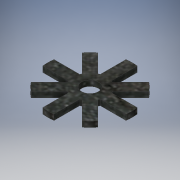
# Autodesk Inventor part: Tooth Disc
Saved by Autodesk Inventor 2019 (Build 230136000, 136)
## iProperties
Created: 2020-01-31
Part Number: Tooth Disc
Material: Steel
Document SubType Name: Modeling
Designer: alb16148
Density: 7.85 g/cm^3
Appearance: Plate
Author: alb16148
Autodesk Inventor part; units mm, degrees
ref_plane "YZ Plane" through (0, 0, 0) normal (1, 0, 0) x (0, 1, 0)
ref_plane "XZ Plane" through (0, 0, 0) normal (0, 1, 0) x (-1, 0, 0)
ref_plane "XY Plane" through (0, 0, 0) normal (0, 0, 1) x (1, 0, 0)
sketch "Sketch1" plane through (0, 0, 0) normal (0, 1, 0) x (-1, 0, 0)
  circle A0 centre (0, 0) radius 3
  circle A1 centre (0, 0) radius 15 construction
  line L0 (14.8661, 2) -> (5.6569, 2)
  line L1 (14.8661, -2) -> (5.6569, -2)
  arc A2 (14.8661, -2) -> (14.8661, 2) centre (0, 0) ccw
  line L2 (9.0977, 11.9261) -> (2.5858, 5.4142)
  arc A3 (11.9261, 9.0977) -> (9.0977, 11.9261) centre (0, 0) ccw
  line L3 (11.9261, 9.0977) -> (5.4142, 2.5858)
  line L4 (-2, 14.8661) -> (-2, 5.6569)
  arc A4 (2, 14.8661) -> (-2, 14.8661) centre (0, 0) ccw
  line L5 (2, 14.8661) -> (2, 5.6569)
  line L6 (-11.9261, 9.0977) -> (-5.4142, 2.5858)
  arc A5 (-9.0977, 11.9261) -> (-11.9261, 9.0977) centre (0, 0) ccw
  line L7 (-9.0977, 11.9261) -> (-2.5858, 5.4142)
  line L8 (-14.8661, -2) -> (-5.6569, -2)
  arc A6 (-14.8661, 2) -> (-14.8661, -2) centre (0, 0) ccw
  line L9 (-14.8661, 2) -> (-5.6569, 2)
  line L10 (-9.0977, -11.9261) -> (-2.5858, -5.4142)
  arc A7 (-11.9261, -9.0977) -> (-9.0977, -11.9261) centre (0, 0) ccw
  line L11 (-11.9261, -9.0977) -> (-5.4142, -2.5858)
  line L12 (2, -14.8661) -> (2, -5.6569)
  arc A8 (-2, -14.8661) -> (2, -14.8661) centre (0, 0) ccw
  line L13 (-2, -14.8661) -> (-2, -5.6569)
  line L14 (11.9261, -9.0977) -> (5.4142, -2.5858)
  arc A9 (9.0977, -11.9261) -> (11.9261, -9.0977) centre (0, 0) ccw
  line L15 (9.0977, -11.9261) -> (2.5858, -5.4142)
  arc A10 (5.4142, -2.5858) -> (5.6569, -2) centre (0, 0) ccw
  arc A11 (2, -5.6569) -> (2.5858, -5.4142) centre (0, 0) ccw
  arc A12 (-2.5858, -5.4142) -> (-2, -5.6569) centre (0, 0) ccw
  arc A13 (-5.6569, -2) -> (-5.4142, -2.5858) centre (0, 0) ccw
  arc A14 (-5.4142, 2.5858) -> (-5.6569, 2) centre (0, 0) ccw
  arc A15 (-2, 5.6569) -> (-2.5858, 5.4142) centre (0, 0) ccw
  arc A16 (5.6569, 2) -> (5.4142, 2.5858) centre (0, 0) ccw
  arc A17 (2.5858, 5.4142) -> (2, 5.6569) centre (0, 0) ccw
  circle A18 centre (0, 0) radius 6 construction
  dimension "d8" = 12
  dimension "d0" = 6
  dimension "d1" = 30
  dimension "d3" = 4
  dimension "d6" = 360
  constraints: 34 point on circle, 32 end point, 18 centre point, 5 coincident, 2 horizontal, 1 vertical alignment, 68 other
  measures "d0" diameter of A0
  measures "d1" diameter of A1
  measures "d3" distance between parallel lines of L1 L0
extrude "Extrusion1" add sketch "Sketch1" along normal blind 2
body "Solid1"
